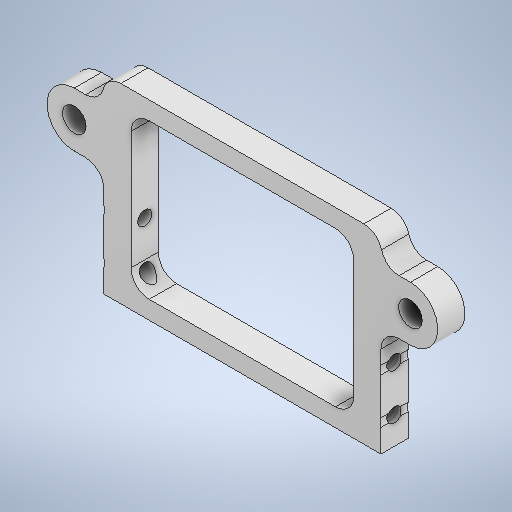
# Autodesk Inventor part: ude_sensor
Saved by Autodesk Inventor 2025.1 (Build 291241000, 241)
## iProperties
Created: 2024-09-09
Part Number: ude_sensor
Material: アルミニウム 2014-T4
Document SubType Name: Modeling
Designer: right
Density: 2.8 g/cm^3
Appearance: サテン
Mass: 2.33454 g
Surface Area: 12.5977 cm^2
Volume: 0.833764 cm^3
Author: right
Autodesk Inventor part; units mm, degrees
ref_plane "YZ Plane" through (0, 0, 0) normal (1, 0, 0) x (0, 1, 0)
ref_plane "XZ Plane" through (0, 0, 0) normal (0, 1, 0) x (-1, 0, 0)
ref_plane "XY Plane" through (0, 0, 0) normal (0, 0, 1) x (1, 0, 0)
sketch "スケッチ1" plane through (0, 0, 0) normal (0, 0, 1) x (1, 0, 0)
  line L0 (0, 0) -> (0, 2.6709) construction
  circle A0 centre (-18.5, 0) radius 1.3
  circle A1 centre (18.5, 0) radius 1.3
  circle A2 centre (-18.5, 0) radius 3
  circle A3 centre (18.5, 0) radius 3
  line L1 (-18.5, 3) -> (18.5, 3)
  line L2 (-18.5, -3) -> (18.5, -3)
  line L3 (-15.25, 6) -> (15.25, 6)
  line L4 (15.25, 6) -> (15.25, -15)
  line L5 (15.25, -15) -> (-15.25, -15)
  line L6 (-15.25, -15) -> (-15.25, 6)
  point P0 (-18.5, 3)
  point P1 (15.25, -3)
  point P2 (-15.25, -3)
  point P3 (-15.25, 3)
  point P4 (15.25, 3)
  point P5 (0, 6)
  point P6 (0, 3)
  dimension "d0" = 2.6
  dimension "d1" = 18.5
  dimension "d2" = 6
  dimension "d3" = 6
  dimension "d6" = 3
  dimension "d7" = 12
  dimension "d9" = 30.5
  constraints: 14 end point, 4 centre point, 4 point on circle, 4 tangent, 2 coincident, 2 midpoint, 2 parallel, 1 horizontal, 1 horizontal alignment, 1 perpendicular, 1 symmetric about line, 1 vertical, 1 vertical alignment, 1 other
  measures "d0" diameter of A0
  measures "d1" distance from line of L0 A0.centre
  measures "d2" diameter of A2
  measures "d3" diameter of A3
  measures "d6" distance from line of L1.end L3
  measures "d7" distance from line of L2.end L5
  measures "d9" distance of L3.start L3.end
extrude "押し出し1" add sketch "スケッチ1" along normal blind 3
fillet "フィレット1" radius 2 6 edges at (-15.25, 3, 1.5) (-15.25, -3, 1.5) (15.25, 3, 1.5) (15.25, -3, 1.5) (-15.25, 6, 1.5) (15.25, 6, 1.5)
sketch "スケッチ4" plane through (0, 0, 0) normal (0, 0, -1) x (-1, 0, 0)
  line L0 (-12.25, 4) -> (12.25, 4)
  line L1 (12.25, 4) -> (12.25, -13)
  line L2 (12.25, -13) -> (-12.25, -13)
  line L3 (-12.25, -13) -> (-12.25, 4)
  line L4 (15.25, -15) -> (-15.25, -15) projected
  line L5 (-13.377, 6) -> (13.377, 6) projected
  line L6 (-15.25, -15) -> (-15.25, -5) projected
  line L7 (15.25, -5) -> (15.25, -15) projected
  point P0 (0, 0)
  dimension "d27" = 2
  dimension "d28" = 2
  dimension "d32" = 3
  dimension "d33" = 3
  constraints: 8 end point, 2 parallel, 1 horizontal, 1 perpendicular
  measures "d27" distance between parallel lines of L4 L2
  measures "d28" distance between parallel lines of L5 L0
  measures "d32" distance between parallel lines of L6 L3
  measures "d33" distance between parallel lines of L1 L7
extrude "押し出し3" cut sketch "スケッチ4" against normal through all
fillet "フィレット2" radius 2 4 edges at (12.25, 4, 1.5) (-12.25, 4, 1.5) (12.25, -13, 1.5) (-12.25, -13, 1.5)
sketch "スケッチ2" plane through (15.25, -15, 3) normal (1, 0, 0) x (0, 0, -1)
  line L0 (3, 0) -> (0, 0) projected
  point P0 (3, 15)
  point P1 (1.5, 3)
  point P2 (1.5, 8)
  point P3 (1.5, 0)
  dimension "d10" = 3
  dimension "d11" = 5
  constraints: 2 vertical alignment, 1 midpoint
  measures "d10" distance from line of L0 point (1.5, 3)
  measures "d11" distance of point (1.5, 3) point (1.5, 8)
hole "穴1" at (15.25, -12, 1.5) at (15.25, -7, 1.5) direction (-1, 0, 0) diameter 1.567 end through all thread size "M2x0.4" class "6H" standard "ISO Metric profile"
sketch "スケッチ3" plane through (0, 0, 3) normal (0, 0, 1) x (1, 0, 0)
  line L0 (-15.25, -12.7835) -> (-15.25, -11.2165) construction
  line L1 (-15.25, -7.7835) -> (-15.25, -6.2165) construction
  line L2 (15.25, -11.2165) -> (15.25, -12.7835) construction
  line L3 (15.25, -6.2165) -> (15.25, -7.7835) construction
  circle A0 centre (-16.25, -12) radius 1.1
  circle A1 centre (-16.25, -7) radius 1.1
  line L4 (-15.25, -15) -> (15.25, -15) construction
  line L5 (0, -15) -> (0, 6) construction
  line L6 (13.377, 6) -> (-13.377, 6) construction
  line L7 (15.25, -12.7835) -> (15.25, -11.2165) construction
  line L8 (15.25, -7.7835) -> (15.25, -6.2165) construction
  circle A2 centre (16.25, -12) radius 1.1
  circle A3 centre (16.25, -7) radius 1.1
  point P0 (0, 0)
  point P1 (-15.25, -12)
  point P2 (-15.25, -7)
  point P3 (15.25, -12)
  point P4 (15.25, -7)
  dimension "d19" = 2.2
  dimension "d20" = 2.2
  dimension "d21" = 1
  dimension "d22" = 1
  constraints: 6 end point, 4 centre point, 4 midpoint, 4 symmetric about line, 2 horizontal alignment, 2 other
  measures "d19" diameter of A0
  measures "d20" diameter of A1
  measures "d21" distance from line of L0 A0.centre
  measures "d22" distance from line of L1 A1.centre
extrude "押し出し2" cut sketch "スケッチ3" against normal through all
